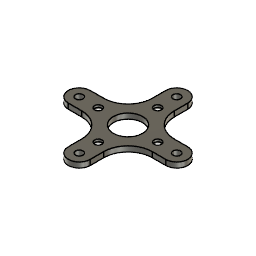
motor-mount (Autodesk Fusion 360 design; units mm, degrees)
part number: 2026-06-20-17-40-02-053
Autodesk Fusion 360 part; units mm, degrees
sketch "Sketch1" plane through (0, 0, 0) normal (0, 0, 1) x (1, 0, 0)
  circle A0 centre (0, 0) radius 164
  line L0 (0, 220) -> (0, -226.5969) construction
  line L1 (-260, 0) -> (224.3647, 0) construction
  circle A1 centre (0, 164) radius 12.5
  line L2 (37, 164) -> (37, 118.79)
  line L3 (-37, 118.79) -> (-37, 164)
  arc A2 (37, 164) -> (-37, 164) centre (0, 164) ccw
  arc A3 (-164, 37) -> (-164, -37) centre (-164, 0) ccw
  circle A4 centre (-164, 0) radius 12.5
  line L4 (-118.79, -37) -> (-164, -37)
  line L5 (-164, 37) -> (-118.79, 37)
  arc A5 (-37, -164) -> (37, -164) centre (0, -164) ccw
  circle A6 centre (0, -164) radius 12.5
  line L6 (37, -118.79) -> (37, -164)
  line L7 (-37, -164) -> (-37, -118.79)
  arc A7 (164, -37) -> (164, 37) centre (164, 0) ccw
  circle A8 centre (164, 0) radius 12.5
  line L8 (118.79, 37) -> (164, 37)
  line L9 (164, -37) -> (118.79, -37)
  arc A9 (37, 118.79) -> (118.79, 37) centre (118.79, 118.79) ccw
  arc A10 (118.79, -37) -> (37, -118.79) centre (118.79, -118.79) ccw
  arc A11 (-37, -118.79) -> (-118.79, -37) centre (-118.79, -118.79) ccw
  arc A12 (-118.79, 37) -> (-37, 118.79) centre (-118.79, 118.79) ccw
  circle A13 centre (100, 0) radius 12.5
  circle A14 centre (0, 100) radius 12.5
  circle A15 centre (-100, 0) radius 12.5
  circle A16 centre (0, -100) radius 12.5
  circle A17 centre (0, 0) radius 49
  dimension "d1" = 328
  dimension "d3" = 74
  dimension "d4" = 25
  dimension "d7" = 45.21
  dimension "d8" = 45.21
  dimension "d10" = 360
  dimension "d11" = 25
  dimension "d12" = 100
  dimension "d14" = 360
  dimension "d15" = 98
  constraint coincident A0.centre A17.centre
  constraint vertical L0
  constraint horizontal L1
  constraint coincident L0 A1.centre
  constraint coincident A0 A1.centre
  constraint concentric A1 A2
  constraint vertical L2
  constraint vertical L3
  constraint tangent L2 A2
  constraint tangent L8 A9
  constraint tangent L2 A9
  constraint tangent L6 A10
  constraint tangent L9 A10
  constraint tangent L4 A11
  constraint tangent L7 A11
  constraint tangent L3 A12
  constraint tangent L5 A12
  constraint coincident L1 A13.centre
  measures "d1" diameter of A0
  measures "d3" diameter of A2
  measures "d4" diameter of A1
  measures "d7" distance of L2.end L2.start
  measures "d8" distance of L3.start L3.end
  measures "d11" diameter of A13
  measures "d12" distance of A0.centre A13.centre
  measures "d15" diameter of A17
extrude "Extrude1" add sketch "Sketch1" along normal blind 18 contours A0 A1 L2 L3 A4 L4 L5 A6 L6 L7 A8 L8 L9 A9 A10 A11 A12 | A0 A7 A8 L8 L9 | A0 A1 L2 L3 A2 | A0 A5 A6 L6 L7 | A0 A3 A4 L4 L5
fillet "Fillet2" radius 10 4 edges at (-111.6541, 4.5202, 0) (-11.6541, -95.4798, 0) (88.3459, 4.5202, 0) (-11.6541, 104.5202, 0)
scale "Scale1" factor 0.5 about (-164, 37, 18) bodies 1
equation "d3 = ( 37 * 2 ) * 1 mm"
